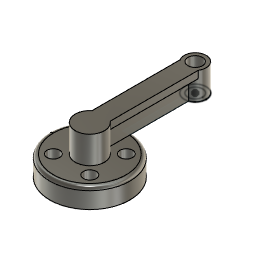
servo_arm (Autodesk Fusion 360 design; units mm, degrees)
Autodesk Fusion 360 part; units mm, degrees
sketch "Aussenscheibe" plane through (0, 0, 0) normal (0, 0, 1) x (1, 0, 0) in component "Servoarm"
  circle A0 centre (0, 0) radius 11
  dimension "d1" = 22
  constraint coincident A0.centre origin
  measures "d1" diameter of A0
extrude "Extrude1" add sketch "Aussenscheibe" along normal blind 5.5 in component "Servoarm"
sketch "Innenscheibe" plane through (0, 0, 0) normal (0, 0, -1) x (1, 0, 0) in component "Servoarm"
  circle A0 centre (0, 0) radius 11
  circle A1 centre (0, 0) radius 10
  dimension "d4" = -1
extrude "Extrude2" cut sketch "Innenscheibe" against normal blind 2 contours A1 in component "Servoarm"
sketch "Scheibenbohrungen" plane through (0, 0, 5.5) normal (0, 0, 1) x (-1, 0, 0) in component "Servoarm"
  circle A0 centre (0, 0) radius 11
  circle A1 centre (5.0205, -5.0205) radius 1.75
  circle A2 centre (5.0205, 5.0205) radius 1.75
  circle A3 centre (-5.0205, 5.0205) radius 1.75
  circle A4 centre (-5.0205, -5.0205) radius 1.75
  dimension "d7" = 3.5
  dimension "d9" = 3.5
  dimension "d11" = 3.5
  dimension "d13" = 3.5
  dimension "d20" = 7.1
  dimension "d21" = 7.1
  dimension "d22" = 7.1
  dimension "d23" = 7.1
  measures "d7" diameter of A1
  measures "d9" diameter of A2
  measures "d11" diameter of A3
  measures "d13" diameter of A4
  measures "d20" distance of A0.centre A1.centre
  measures "d21" distance of A0.centre A4.centre
  measures "d22" distance of A0.centre A3.centre
  measures "d23" distance of A0.centre A2.centre
extrude "Extrude3" cut sketch "Scheibenbohrungen" against normal up to surface (3.5 mm away) contours A1 | A2 | A3 | A4 in component "Servoarm"
sketch "Schraubenkopf" plane through (0, 0, 2) normal (0, 0, -1) x (1, 0, 0) in component "Servoarm"
  circle A0 centre (5.0205, 5.0205) radius 1.75
  circle A1 centre (-5.0205, 5.0205) radius 1.75
  circle A2 centre (5.0205, -5.0205) radius 1.75
  circle A3 centre (-5.0205, -5.0205) radius 1.75
  circle A4 centre (0, 0) radius 10
  circle A5 centre (0, 0) radius 2.75
  dimension "d17" = 5.5
  constraint coincident A4.centre A5.centre
  measures "d17" diameter of A5
extrude "Extrude4" cut sketch "Schraubenkopf" against normal blind 1.5 contours A5 in component "Servoarm"
sketch "Aushebung" plane through (0, 0, 5.5) normal (0, 0, 1) x (-1, 0, 0) in component "Servoarm"
  circle A0 centre (-5.0205, 5.0205) radius 1.75
  circle A1 centre (5.0205, 5.0205) radius 1.75
  circle A2 centre (-5.0205, -5.0205) radius 1.75
  circle A3 centre (5.0205, -5.0205) radius 1.75
  circle A4 centre (0, 0) radius 11
  circle A5 centre (0, 0) radius 4
  dimension "d24" = 8
  constraint coincident A4.centre A5.centre
  measures "d24" diameter of A5
extrude "Extrude5" add sketch "Aushebung" along normal blind 7.5 contours A5 in component "Servoarm"
fillet "Fillet1" radius 1 curvature continuous 1 edges at (-10.2556, -3.9778, 5.5) in component "Servoarm"
ref_plane "WorkPlane1" through (0, 4, 9.2522) normal (0, 1, 0) x (1, 0, 0) in component "Servoarm"
sketch "Armprofil" plane through (0, 4, 9.2522) normal (0, 1, 0) x (1, 0, 0) in component "Servoarm"
  line L0 (-4, -3.7478) -> (4, -3.7478)
  line L1 (-4, -3.7478) -> (4, -3.7478)
  line L2 (4, 3.7522) -> (-4, 3.7522)
  line L3 (1, -1.7478) -> (1, 3.7522)
  line L4 (0, 3.7522) -> (1, 3.7522)
  line L5 (0, 3.7522) -> (0, -3.7478)
  line L6 (0, -3.7478) -> (2.5, -3.7478) construction
  line L7 (2.5, -1.7478) -> (1, -1.7478)
  line L8 (2.5, -3.7478) -> (2.5, -1.7478)
  line L9 (0, -3.7478) -> (-2.5, -3.7478) construction
  line L10 (-2.5, -3.7478) -> (-2.5, -1.7478)
  line L11 (-2.5, -1.7478) -> (-1, -1.7478)
  line L12 (0, 3.7522) -> (-1, 3.7522)
  line L13 (-1, -1.7478) -> (-1, 3.7522)
  dimension "d34" = 2.5
  dimension "d35" = 1
  dimension "d36" = 2
  constraint midpoint L1 L5.end
  constraint coincident L2 L3.end
  constraint perpendicular L2 L3
  constraint midpoint L2 L4.start
  constraint coincident L0 L6.end
  constraint perpendicular L5 L6
  constraint perpendicular L3 L7
  constraint perpendicular L7 L8
  constraint symmetric L6.start L5 L9.start
  constraint symmetric L3.start L5 L11.end
  constraint symmetric L3.end L5 L12.end
  constraint symmetric L4.start L5 L12.start
  constraint symmetric L5 L6.end L9.end
  constraint symmetric L5 L7.start L10.end
  measures "d34" distance of L5.end L6.end
  measures "d35" distance of L3.end L4.start
  measures "d36" distance of L6.end L7.start
extrude "Extrude7" add sketch "Armprofil" against normal blind 4 in component "Servoarm"
extrude "Extrude8" add 1 faces at (0.3333, 4, 12.3333) along direction (0, 1, 0) blind 25 in component "Servoarm"
sketch "Sketch8" plane through (0, 0, 5.5) normal (0, 0, -1) x (1, 0, 0) in component "Servoarm"
  arc A0 (-1, -9.9499) -> (1, -9.9499) centre (0, 0) ccw
  line L0 (-1, -9.9499) -> (-1, -29)
  line L1 (-1, -29) -> (1, -29)
  line L2 (1, -29) -> (1, -9.9499)
  circle A1 centre (0, -29) radius 3
  circle A2 centre (0, -29) radius 2
  dimension "d46" = 6
  dimension "d47" = -1
  constraint midpoint L1 A1.centre
  measures "d46" diameter of A1
extrude "Extrude9" add sketch "Sketch8" against normal up to surface (7.5 mm away) contours L0 L2 A1 A2 picked at (-2.543, -29.7849) in component "Servoarm"
extrude "Extrude10" cut sketch "Sketch8" against normal up to surface (7.5 mm away) contours L0 L1 L2 A2 | L0 L1 L2 A2 in component "Servoarm"
component "Servoarm" placed x (1, 0, 0) y (0, 1, 0) z (0, 0, 1) at (0, 0, 0)
